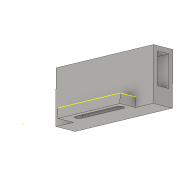
# Autodesk Inventor part: OPB732_CASE_BOTTOM
Saved by Autodesk Inventor 2016 (Build 200138000, 138)
## iProperties
Created: 2015-05-25
Part Number: OPB732_CASE_BOTTOM
Material: Generic
Document SubType Name: Modeling
Designer: Admin
Density: 1 g/cm^3
Appearance: Default
Author: Admin
Autodesk Inventor part; units mm, degrees
ref_plane "YZ Plane" through (0, 0, 0) normal (1, 0, 0) x (0, 1, 0)
ref_plane "XZ Plane" through (0, 0, 0) normal (0, 1, 0) x (-1, 0, 0)
ref_plane "XY Plane" through (0, 0, 0) normal (0, 0, 1) x (1, 0, 0)
sketch "Skizze14" plane through (0, 0, 0) normal (0, 1, 0) x (-1, 0, 0)
  line L0 (0, 0) -> (28, 0)
  line L1 (28, 0) -> (28, 67)
  line L2 (28, 67) -> (0, 67)
  line L3 (0, 67) -> (0, 0)
  dimension "d40" = 28
  dimension "d41" = 67
  constraints: 8 end point, 2 parallel, 1 horizontal, 1 perpendicular
  measures "d40" distance of L2.end L1.end
  measures "d41" distance of L1.end L0.end
extrude "Extrusion13" add sketch "Skizze14" along normal blind 10
sketch "Skizze15" plane through (-28, 0, 67) normal (0, 0, 1) x (1, 0, 0)
  line L0 (2, 8) -> (15, 8)
  line L1 (15, 8) -> (15, 2)
  line L2 (15, 2) -> (2, 2)
  line L3 (2, 2) -> (2, 8)
  dimension "d44" = 13
  dimension "d45" = 6
  constraints: 8 end point, 2 parallel, 1 horizontal, 1 perpendicular
  measures "d44" distance of L1.end L2.end
  measures "d45" distance of L0.end L1.end
extrude "Extrusion14" cut sketch "Skizze15" against normal blind 13
sketch "Skizze16" plane through (-28, 0, 54) normal (0, 0, 1) x (1, 0, 0)
  line L0 (3, 8) -> (14, 8)
  line L1 (14, 8) -> (14, 3)
  line L2 (14, 3) -> (3, 3)
  line L3 (3, 3) -> (3, 8)
  point P0 (28, 0)
  constraints: 8 end point, 2 parallel, 1 horizontal, 1 perpendicular
extrude "Extrusion15" cut sketch "Skizze16" against normal blind 60
sketch "Skizze21" plane through (0, 0, 0) normal (0, 0, -1) x (-1, 0, 0)
  line L0 (25, 8) -> (25, 3) projected
  line L1 (25, 3) -> (14, 3) projected
  line L2 (14, 3) -> (14, 8) projected
  line L3 (14, 8) -> (25, 8) projected
  line L4 (0, 0) -> (28, 0) projected
  line L5 (28, 0) -> (28, 10) projected
  line L6 (28, 10) -> (0, 10)
  line L7 (0, 10) -> (0, 0)
  line L8 (0, 0) -> (28, 0)
  line L9 (28, 0) -> (28, 10)
  constraints: 8 end point, 2 parallel, 1 horizontal, 1 perpendicular
extrude "Extrusion20" cut sketch "Skizze21" against normal blind 17
sketch "Skizze23" plane through (-28, 0, 67) normal (0, 0, 1) x (1, 0, 0)
  line L0 (28, 0) -> (28, 10) projected
  line L1 (28, 0) -> (22, 0)
  line L2 (22, 0) -> (22, 10)
  line L3 (22, 10) -> (28, 10)
  line L4 (28, 10) -> (28, 0)
  constraints: 8 end point, 2 parallel, 1 horizontal, 1 perpendicular
extrude "Extrusion22" cut sketch "Skizze23" against normal blind 60
sketch "Skizze24" plane through (0, 0, 0) normal (0, -1, 0) x (1, 0, 0)
  line L0 (-6, 17) -> (-6, 67) projected
  line L1 (-10, 26) -> (-6, 26)
  line L2 (-6, 26) -> (-6, 58)
  line L3 (-6, 58) -> (-10, 58)
  line L4 (-10, 58) -> (-10, 26)
  point P0 (0, 0)
  constraints: 8 end point, 2 parallel, 1 horizontal, 1 perpendicular, 1 point on line
extrude "Extrusion23" add sketch "Skizze24" along normal blind 8
sketch "Skizze25" plane through (-10, 0, 26) normal (-1, 0, 0) x (0, 0, 1)
  line L0 (0, 0) -> (0, -8) projected
  line L1 (7, -4) -> (28, -4) construction
  line L2 (7, -5.75) -> (28, -5.75)
  line L3 (28, -2.25) -> (7, -2.25)
  arc A0 (7, -2.25) -> (7, -5.75) centre (7, -4) ccw
  arc A1 (28, -5.75) -> (28, -2.25) centre (28, -4) ccw
  point P0 (-26, 0)
  point P1 (17.5, -4)
  dimension "d70" = 3.5
  constraints: 8 end point, 4 point on circle, 4 tangent, 2 centre point, 1 midpoint, 1 parallel, 1 perpendicular
  measures "d70" diameter of A1
extrude "Extrusion24" cut sketch "Skizze25" against normal blind 12
sketch "Skizze26" plane through (-10, 0, 26) normal (-1, 0, 0) x (0, 0, 1)
  arc A0 (28, -5.75) -> (28, -2.25) centre (28, -4) ccw projected
  line L0 (28, -5.75) -> (7, -5.75) projected
  arc A1 (7, -2.25) -> (7, -5.75) centre (7, -4) ccw projected
  line L1 (7, -2.25) -> (28, -2.25) projected
  line L2 (0, 0) -> (32, 0) projected
  line L3 (0, 0) -> (0, -8) projected
  line L4 (32, -8) -> (0, -8) projected
  line L5 (32, 0) -> (32, -8) projected
  point P0 (-26, 0)
